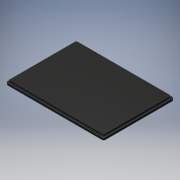
# Autodesk Inventor part: receiver-box-lid
Saved by Autodesk Inventor 2017 (Build 210142000, 142)
## iProperties
Created: 2020-06-15
Part Number: receiver-box-lid
Material: ABS Plastic
Document SubType Name: Modeling
Designer: HAYNIE R&D
Density: 1.06 g/cm^3
Appearance: Glossy - Black
Author: HAYNIE R&D
Autodesk Inventor part; units mm, degrees
(part 1 of 2)
ref_plane "YZ Plane" through (0, 0, 0) normal (1, 0, 0) x (0, 1, 0)
ref_plane "XZ Plane" through (0, 0, 0) normal (0, 1, 0) x (-1, 0, 0)
ref_plane "XY Plane" through (0, 0, 0) normal (0, 0, 1) x (1, 0, 0)
sketch "Sketch2" plane through (0, 0, 0) normal (0, 1, 0) x (-1, 0, 0)
  line L0 (0.0012, 0.0002) -> (-124.9988, 0.0002)
  line L1 (-124.9988, 0.0002) -> (-124.9988, -89.9998)
  line L2 (-124.9988, -89.9998) -> (0.0012, -89.9998)
  line L3 (0.0012, -89.9998) -> (0.0012, 0.0002)
  point P0 (0, 0)
  dimension "d1" = 125
  dimension "d2" = 90
  constraints: 8 end point, 2 parallel, 1 horizontal, 1 perpendicular
  measures "d1" distance of L2.end L1.end
  measures "d2" distance of L1.end L0.end
extrude "Extrusion1" add sketch "Sketch2" along normal blind 2.5
sketch "Sketch3" plane through (0, 2.5, 0) normal (0, 1, 0) x (1, 0, 0)
  line L0 (1.9988, 87.9998) -> (122.9988, 87.9998)
  line L1 (122.9988, 87.9998) -> (122.9988, 1.9998)
  line L2 (122.9988, 1.9998) -> (1.9988, 1.9998)
  line L3 (1.9988, 1.9998) -> (1.9988, 87.9998)
  line L4 (-0.0012, -0.0002) -> (124.9988, -0.0002) projected
  line L5 (124.9988, 89.9998) -> (-0.0012, 89.9998) projected
  line L6 (124.9988, -0.0002) -> (124.9988, 89.9998) projected
  line L7 (-0.0012, 89.9998) -> (-0.0012, -0.0002) projected
  point P0 (0, 0)
  dimension "d13" = 2
  dimension "d14" = 2
  dimension "d15" = 2
  dimension "d16" = 2
  constraints: 8 end point, 2 parallel, 1 horizontal, 1 perpendicular
  measures "d13" distance between parallel lines of L4 L2
  measures "d14" distance between parallel lines of L5 L0
  measures "d15" distance between parallel lines of L1 L6
  measures "d16" distance between parallel lines of L7 L3
extrude "Extrusion2" add sketch "Sketch3" along normal blind 2.5 contours L0 L1 L2 L3
fillet "Fillet1" radius 2 1 edges at (-0.0012, 1.25, 0.0002)
fillet "Fillet2" radius 2 1 edges at (124.9988, 1.25, 0.0002)
fillet "Fillet3" radius 2 1 edges at (124.9988, 1.25, -89.9998)
fillet "Fillet4" radius 2 1 edges at (-0.0012, 1.25, -89.9998)
fillet "Fillet5" radius 2 1 edges at (122.9988, 3.75, -1.9998)
fillet "Fillet6" radius 2 1 edges at (122.9988, 3.75, -87.9998)
fillet "Fillet7" radius 2 1 edges at (1.9988, 3.75, -87.9998)
sketch "Sketch4" plane through (0, 0, 0) normal (0, -1, 0) x (1, 0, 0)
  line L0 (-6.3841, 4.5799) -> (131.1521, 4.5799) construction
  line L1 (131.1521, 4.5799) -> (131.1521, -94.6516) construction
  line L2 (131.1521, -94.6516) -> (-6.3841, -94.6516) construction
  line L3 (-6.3841, -94.6516) -> (-6.3841, 4.5799) construction
  line L4 (20.0195, -41.0232) -> (19.5544, -41.0232)
  line L5 (19.5544, -41.0232) -> (19.5544, -39.3101)
  line L6 (19.5544, -39.3101) -> (17.9434, -39.3101)
  line L7 (17.9434, -39.3101) -> (17.9434, -41.0232)
  line L8 (17.9434, -41.0232) -> (17.4782, -41.0232)
  line L9 (17.4782, -41.0232) -> (17.4782, -37.5232)
  line L10 (17.4782, -37.5232) -> (17.9434, -37.5232)
  line L11 (17.9434, -37.5232) -> (17.9434, -38.896)
  line L12 (17.9434, -38.896) -> (19.5544, -38.896)
  line L13 (19.5544, -38.896) -> (19.5544, -37.5232)
  line L14 (19.5544, -37.5232) -> (20.0195, -37.5232)
  line L15 (20.0195, -37.5232) -> (20.0195, -41.0232)
  line L16 (20.3514, -41.0232) -> (21.5313, -37.5232)
  line L17 (21.5313, -37.5232) -> (22.1042, -37.5232)
  line L18 (22.1042, -37.5232) -> (23.2841, -41.0232)
  line L19 (23.2841, -41.0232) -> (22.7934, -41.0232)
  line L20 (22.7934, -41.0232) -> (22.4758, -40.0447)
  line L21 (22.4758, -40.0447) -> (21.1399, -40.0447)
  line L22 (21.1399, -40.0447) -> (20.8222, -41.0232)
  line L23 (20.8222, -41.0232) -> (20.3514, -41.0232)
  line L24 (22.3481, -39.6476) -> (21.8064, -37.9997)
  line L25 (21.8064, -37.9997) -> (21.2675, -39.6476)
  line L26 (21.2675, -39.6476) -> (22.3481, -39.6476)
  line L27 (26.0665, -37.5232) -> (24.8838, -39.4746)
  line L28 (24.8838, -39.4746) -> (24.8838, -41.0232)
  line L29 (24.8838, -41.0232) -> (24.4187, -41.0232)
  line L30 (24.4187, -41.0232) -> (24.4187, -39.5228)
  line L31 (24.4187, -39.5228) -> (23.2359, -37.5232)
  line L32 (23.2359, -37.5232) -> (23.7521, -37.5232)
  line L33 (23.7521, -37.5232) -> (24.6541, -39.0633)
  line L34 (24.6541, -39.0633) -> (25.573, -37.5232)
  line L35 (25.573, -37.5232) -> (26.0665, -37.5232)
  line L36 (28.8943, -41.0232) -> (28.3725, -41.0232)
  line L37 (28.3725, -41.0232) -> (26.8238, -38.0054)
  line L38 (26.8238, -38.0054) -> (26.8238, -41.0232)
  line L39 (26.8238, -41.0232) -> (26.3899, -41.0232)
  line L40 (26.3899, -41.0232) -> (26.3899, -37.5232)
  line L41 (26.3899, -37.5232) -> (27.0507, -37.5232)
  line L42 (27.0507, -37.5232) -> (28.4604, -40.2943)
  line L43 (28.4604, -40.2943) -> (28.4604, -37.5232)
  line L44 (28.4604, -37.5232) -> (28.8943, -37.5232)
  line L45 (28.8943, -37.5232) -> (28.8943, -41.0232)
  line L46 (30.823, -41.0232) -> (29.4673, -41.0232)
  line L47 (29.4673, -41.0232) -> (29.4673, -40.6658)
  line L48 (29.4673, -40.6658) -> (29.9126, -40.6658)
  line L49 (29.9126, -40.6658) -> (29.9126, -37.8806)
  line L50 (29.9126, -37.8806) -> (29.4673, -37.8806)
  line L51 (29.4673, -37.8806) -> (29.4673, -37.5232)
  line L52 (29.4673, -37.5232) -> (30.823, -37.5232)
  line L53 (30.823, -37.5232) -> (30.823, -37.8806)
  line L54 (30.823, -37.8806) -> (30.3777, -37.8806)
  line L55 (30.3777, -37.8806) -> (30.3777, -40.6658)
  line L56 (30.3777, -40.6658) -> (30.823, -40.6658)
  line L57 (30.823, -40.6658) -> (30.823, -41.0232)
  line L58 (31.3988, -41.0232) -> (31.3988, -37.5232)
  line L59 (31.3988, -37.5232) -> (33.5884, -37.5232)
  line L60 (33.5884, -37.5232) -> (33.5884, -37.9373)
  line L61 (33.5884, -37.9373) -> (31.8639, -37.9373)
  line L62 (31.8639, -37.9373) -> (31.8639, -38.896)
  line L63 (31.8639, -38.896) -> (33.4721, -38.896)
  line L64 (33.4721, -38.896) -> (33.4721, -39.3101)
  line L65 (33.4721, -39.3101) -> (31.8639, -39.3101)
  line L66 (31.8639, -39.3101) -> (31.8639, -40.6091)
  line L67 (31.8639, -40.6091) -> (33.5884, -40.6091)
  line L68 (33.5884, -40.6091) -> (33.5884, -41.0232)
  line L69 (33.5884, -41.0232) -> (31.3988, -41.0232)
  line L70 (38.3109, -41.0232) -> (37.7067, -41.0232)
  line L71 (37.7067, -41.0232) -> (36.6006, -39.6306)
  line L72 (36.6006, -39.6306) -> (36.0674, -39.6306)
  line L73 (36.0674, -39.6306) -> (36.0674, -41.0232)
  line L74 (36.0674, -41.0232) -> (35.6022, -41.0232)
  line L75 (35.6022, -41.0232) -> (35.6022, -37.5232)
  line L76 (35.6022, -37.5232) -> (36.5041, -37.5232)
  spline S0 degree 2 poles (36.5041, -37.5232) (36.8048, -37.5232) (37.2104, -37.5884) (37.3947, -37.7075) knots 0 0 0 1 2 2 2
  spline S1 degree 2 poles (37.3947, -37.7075) (37.5791, -37.8267) (37.7918, -38.1982) (37.7918, -38.4733) knots 0 0 0 1 2 2 2
  spline S2 degree 2 poles (37.7918, -38.4733) (37.7918, -38.8562) (37.4004, -39.3753) (37.0657, -39.5001) knots 0 0 0 1 2 2 2
  line L77 (37.0657, -39.5001) -> (38.3109, -41.0232)
  spline S3 degree 2 poles (37.3068, -38.5102) (37.3068, -38.3571) (37.199, -38.1216) (37.0856, -38.0451) knots 0 0 0 1 2 2 2
  spline S4 degree 2 poles (37.0856, -38.0451) (36.9863, -37.9798) (36.7225, -37.9259) (36.5297, -37.9259) knots 0 0 0 1 2 2 2
  line L78 (36.5297, -37.9259) -> (36.0674, -37.9259)
  line L79 (36.0674, -37.9259) -> (36.0674, -39.242)
  line L80 (36.0674, -39.242) -> (36.4758, -39.242)
  spline S5 degree 2 poles (36.4758, -39.242) (36.6772, -39.242) (36.9977, -39.1711) (37.1083, -39.0605) knots 0 0 0 1 2 2 2
  spline S6 degree 2 poles (37.1083, -39.0605) (37.2104, -38.964) (37.3068, -38.6917) (37.3068, -38.5102) knots 0 0 0 1 2 2 2
  line L81 (38.5888, -41.0232) -> (38.5888, -37.5232)
  line L82 (38.5888, -37.5232) -> (40.7785, -37.5232)
  line L83 (40.7785, -37.5232) -> (40.7785, -37.9373)
  line L84 (40.7785, -37.9373) -> (39.054, -37.9373)
  line L85 (39.054, -37.9373) -> (39.054, -38.896)
  line L86 (39.054, -38.896) -> (40.6622, -38.896)
  line L87 (40.6622, -38.896) -> (40.6622, -39.3101)
  line L88 (40.6622, -39.3101) -> (39.054, -39.3101)
  line L89 (39.054, -39.3101) -> (39.054, -40.6091)
  line L90 (39.054, -40.6091) -> (40.7785, -40.6091)
  line L91 (40.7785, -40.6091) -> (40.7785, -41.0232)
  line L92 (40.7785, -41.0232) -> (38.5888, -41.0232)
  spline S7 degree 2 poles (42.2647, -41.0856) (41.8846, -41.0856) (41.3514, -40.9267) (41.116, -40.8133) knots 0 0 0 1 2 2 2
  line L93 (41.116, -40.8133) -> (41.116, -40.229)
  line L94 (41.116, -40.229) -> (41.15, -40.229)
  spline S8 degree 2 poles (41.15, -40.229) (41.3798, -40.4446) (41.9612, -40.6828) (42.2306, -40.6828) knots 0 0 0 1 2 2 2
  spline S9 degree 2 poles (42.2306, -40.6828) (42.6164, -40.6828) (43.0106, -40.3623) (43.0106, -40.0985) knots 0 0 0 1 2 2 2
  spline S10 degree 2 poles (43.0106, -40.0985) (43.0106, -39.8887) (42.8036, -39.6277) (42.5795, -39.5625) knots 0 0 0 1 2 2 2
  spline S11 degree 2 poles (42.5795, -39.5625) (42.4178, -39.5171) (42.1484, -39.4547) (41.947, -39.4037) knots 0 0 0 1 2 2 2
  spline S12 degree 2 poles (41.947, -39.4037) (41.7655, -39.3554) (41.479, -39.2108) (41.3684, -39.0945) knots 0 0 0 1 2 2 2
  spline S13 degree 2 poles (41.3684, -39.0945) (41.2606, -38.9782) (41.1415, -38.6662) (41.1415, -38.462) knots 0 0 0 1 2 2 2
  spline S14 degree 2 poles (41.1415, -38.462) (41.1415, -38.0366) (41.8052, -37.4608) (42.3186, -37.4608) knots 0 0 0 1 2 2 2
  spline S15 degree 2 poles (42.3186, -37.4608) (42.6135, -37.4608) (43.1354, -37.5771) (43.3595, -37.6877) knots 0 0 0 1 2 2 2
  line L95 (43.3595, -37.6877) -> (43.3595, -38.2436)
  line L96 (43.3595, -38.2436) -> (43.3255, -38.2436)
  spline S16 degree 2 poles (43.3255, -38.2436) (43.1581, -38.0904) (42.6362, -37.8635) (42.3498, -37.8635) knots 0 0 0 1 2 2 2
  spline S17 degree 2 poles (42.3498, -37.8635) (42.0264, -37.8635) (41.6265, -38.167) (41.6265, -38.4138) knots 0 0 0 1 2 2 2
  spline S18 degree 2 poles (41.6265, -38.4138) (41.6265, -38.635) (41.8619, -38.8988) (42.0832, -38.9584) knots 0 0 0 1 2 2 2
  spline S19 degree 2 poles (42.0832, -38.9584) (42.2306, -38.9981) (42.6589, -39.1002) (42.8007, -39.1427) knots 0 0 0 1 2 2 2
  spline S20 degree 2 poles (42.8007, -39.1427) (43.161, -39.2533) (43.4956, -39.6986) (43.4956, -40.0248) knots 0 0 0 1 2 2 2
  spline S21 degree 2 poles (43.4956, -40.0248) (43.4956, -40.2319) (43.3283, -40.6289) (43.178, -40.7679) knots 0 0 0 1 2 2 2
  spline S22 degree 2 poles (43.178, -40.7679) (43.0106, -40.9211) (42.5852, -41.0856) (42.2647, -41.0856) knots 0 0 0 1 2 2 2
  line L97 (43.9693, -41.0232) -> (43.9693, -37.5232)
  line L98 (43.9693, -37.5232) -> (46.1589, -37.5232)
  line L99 (46.1589, -37.5232) -> (46.1589, -37.9373)
  line L100 (46.1589, -37.9373) -> (44.4345, -37.9373)
  line L101 (44.4345, -37.9373) -> (44.4345, -38.896)
  line L102 (44.4345, -38.896) -> (46.0426, -38.896)
  line L103 (46.0426, -38.896) -> (46.0426, -39.3101)
  line L104 (46.0426, -39.3101) -> (44.4345, -39.3101)
  line L105 (44.4345, -39.3101) -> (44.4345, -40.6091)
  line L106 (44.4345, -40.6091) -> (46.1589, -40.6091)
  line L107 (46.1589, -40.6091) -> (46.1589, -41.0232)
  line L108 (46.1589, -41.0232) -> (43.9693, -41.0232)
  line L109 (46.2922, -41.0232) -> (47.4721, -37.5232)
  line L110 (47.4721, -37.5232) -> (48.0451, -37.5232)
  line L111 (48.0451, -37.5232) -> (49.225, -41.0232)
  line L112 (49.225, -41.0232) -> (48.7343, -41.0232)
  line L113 (48.7343, -41.0232) -> (48.4166, -40.0447)
  line L114 (48.4166, -40.0447) -> (47.0807, -40.0447)
  line L115 (47.0807, -40.0447) -> (46.7631, -41.0232)
  line L116 (46.7631, -41.0232) -> (46.2922, -41.0232)
  line L117 (48.289, -39.6476) -> (47.7473, -37.9997)
  line L118 (47.7473, -37.9997) -> (47.2084, -39.6476)
  line L119 (47.2084, -39.6476) -> (48.289, -39.6476)
  line L120 (52.2655, -41.0232) -> (51.6614, -41.0232)
  line L121 (51.6614, -41.0232) -> (50.5552, -39.6306)
  line L122 (50.5552, -39.6306) -> (50.022, -39.6306)
  line L123 (50.022, -39.6306) -> (50.022, -41.0232)
  line L124 (50.022, -41.0232) -> (49.5568, -41.0232)
  line L125 (49.5568, -41.0232) -> (49.5568, -37.5232)
  line L126 (49.5568, -37.5232) -> (50.4588, -37.5232)
  spline S23 degree 2 poles (50.4588, -37.5232) (50.7594, -37.5232) (51.165, -37.5884) (51.3494, -37.7075) knots 0 0 0 1 2 2 2
  spline S24 degree 2 poles (51.3494, -37.7075) (51.5337, -37.8267) (51.7464, -38.1982) (51.7464, -38.4733) knots 0 0 0 1 2 2 2
  spline S25 degree 2 poles (51.7464, -38.4733) (51.7464, -38.8562) (51.355, -39.3753) (51.0204, -39.5001) knots 0 0 0 1 2 2 2
  line L127 (51.0204, -39.5001) -> (52.2655, -41.0232)
  spline S26 degree 2 poles (51.2614, -38.5102) (51.2614, -38.3571) (51.1537, -38.1216) (51.0402, -38.0451) knots 0 0 0 1 2 2 2
  spline S27 degree 2 poles (51.0402, -38.0451) (50.9409, -37.9798) (50.6772, -37.9259) (50.4843, -37.9259) knots 0 0 0 1 2 2 2
  line L128 (50.4843, -37.9259) -> (50.022, -37.9259)
  line L129 (50.022, -37.9259) -> (50.022, -39.242)
  line L130 (50.022, -39.242) -> (50.4304, -39.242)
  spline S28 degree 2 poles (50.4304, -39.242) (50.6318, -39.242) (50.9523, -39.1711) (51.0629, -39.0605) knots 0 0 0 1 2 2 2
  spline S29 degree 2 poles (51.0629, -39.0605) (51.165, -38.964) (51.2614, -38.6917) (51.2614, -38.5102) knots 0 0 0 1 2 2 2
  spline S30 degree 2 poles (53.9105, -41.0856) (53.5702, -41.0856) (52.9944, -40.8558) (52.7845, -40.6261) knots 0 0 0 1 2 2 2
  spline S31 degree 2 poles (52.7845, -40.6261) (52.5746, -40.3992) (52.3449, -39.7185) (52.3449, -39.276) knots 0 0 0 1 2 2 2
  spline S32 degree 2 poles (52.3449, -39.276) (52.3449, -38.8364) (52.569, -38.184) (52.7817, -37.943) knots 0 0 0 1 2 2 2
  spline S33 degree 2 poles (52.7817, -37.943) (52.9916, -37.7075) (53.5645, -37.4608) (53.9191, -37.4608) knots 0 0 0 1 2 2 2
  spline S34 degree 2 poles (53.9191, -37.4608) (54.0949, -37.4608) (54.4041, -37.5118) (54.5345, -37.5515) knots 0 0 0 1 2 2 2
  spline S35 degree 2 poles (54.5345, -37.5515) (54.648, -37.5884) (54.8834, -37.6934) (54.9997, -37.7558) knots 0 0 0 1 2 2 2
  line L131 (54.9997, -37.7558) -> (54.9997, -38.3173)
  line L132 (54.9997, -38.3173) -> (54.9628, -38.3173)
  spline S36 degree 2 poles (54.9628, -38.3173) (54.9004, -38.2606) (54.7075, -38.1018) (54.5686, -38.0252) knots 0 0 0 1 2 2 2
  spline S37 degree 2 poles (54.5686, -38.0252) (54.4353, -37.9515) (54.1204, -37.8579) (53.9162, -37.8579) knots 0 0 0 1 2 2 2
  spline S38 degree 2 poles (53.9162, -37.8579) (53.6922, -37.8579) (53.2922, -38.0422) (53.1419, -38.2181) knots 0 0 0 1 2 2 2
  spline S39 degree 2 poles (53.1419, -38.2181) (52.9944, -38.3968) (52.8299, -38.9385) (52.8299, -39.276) knots 0 0 0 1 2 2 2
  spline S40 degree 2 poles (52.8299, -39.276) (52.8299, -39.6362) (53.0029, -40.1553) (53.1533, -40.334) knots 0 0 0 1 2 2 2
  spline S41 degree 2 poles (53.1533, -40.334) (53.3007, -40.507) (53.695, -40.6828) (53.9162, -40.6828) knots 0 0 0 1 2 2 2
  spline S42 degree 2 poles (53.9162, -40.6828) (54.1176, -40.6828) (54.4608, -40.5836) (54.5941, -40.5098) knots 0 0 0 1 2 2 2
  spline S43 degree 2 poles (54.5941, -40.5098) (54.7217, -40.4361) (54.9118, -40.2829) (54.9657, -40.229) knots 0 0 0 1 2 2 2
  line L133 (54.9657, -40.229) -> (54.9997, -40.229)
  line L134 (54.9997, -40.229) -> (54.9997, -40.7849)
  spline S44 degree 2 poles (54.9997, -40.7849) (54.8834, -40.8388) (54.6792, -40.9381) (54.5345, -40.9835) knots 0 0 0 1 2 2 2
  spline S45 degree 2 poles (54.5345, -40.9835) (54.3814, -41.0345) (54.1204, -41.0856) (53.9105, -41.0856) knots 0 0 0 1 2 2 2
  line L135 (57.975, -41.0232) -> (57.5098, -41.0232)
  line L136 (57.5098, -41.0232) -> (57.5098, -39.3101)
  line L137 (57.5098, -39.3101) -> (55.8988, -39.3101)
  line L138 (55.8988, -39.3101) -> (55.8988, -41.0232)
  line L139 (55.8988, -41.0232) -> (55.4336, -41.0232)
  line L140 (55.4336, -41.0232) -> (55.4336, -37.5232)
  line L141 (55.4336, -37.5232) -> (55.8988, -37.5232)
  line L142 (55.8988, -37.5232) -> (55.8988, -38.896)
  line L143 (55.8988, -38.896) -> (57.5098, -38.896)
  line L144 (57.5098, -38.896) -> (57.5098, -37.5232)
  line L145 (57.5098, -37.5232) -> (57.975, -37.5232)
  line L146 (57.975, -37.5232) -> (57.975, -41.0232)
  line L147 (63.2278, -41.0232) -> (62.6265, -41.0232)
  line L148 (62.6265, -41.0232) -> (62.1472, -40.5212)
  spline S46 degree 2 poles (62.1472, -40.5212) (61.9089, -40.8275) (61.4041, -41.0969) (61.0836, -41.0969) knots 0 0 0 1 2 2 2
  spline S47 degree 2 poles (61.0836, -41.0969) (60.6099, -41.0969) (59.9916, -40.524) (59.9916, -40.0617) knots 0 0 0 1 2 2 2
  spline S48 degree 2 poles (59.9916, -40.0617) (59.9916, -39.8603) (60.105, -39.5455) (60.1986, -39.4178) knots 0 0 0 1 2 2 2
  spline S49 degree 2 poles (60.1986, -39.4178) (60.2894, -39.2959) (60.5305, -39.1087) (60.6383, -39.0406) knots 0 0 0 1 2 2 2
  spline S50 degree 2 poles (60.6383, -39.0406) (60.4028, -38.8818) (60.1674, -38.5272) (60.1674, -38.2606) knots 0 0 0 1 2 2 2
  spline S51 degree 2 poles (60.1674, -38.2606) (60.1674, -38.0933) (60.3007, -37.8097) (60.4085, -37.7019) knots 0 0 0 1 2 2 2
  spline S52 degree 2 poles (60.4085, -37.7019) (60.522, -37.5913) (60.8822, -37.4494) (61.0949, -37.4494) knots 0 0 0 1 2 2 2
  spline S53 degree 2 poles (61.0949, -37.4494) (61.4863, -37.4494) (61.9798, -37.8607) (61.9798, -38.1755) knots 0 0 0 1 2 2 2
  spline S54 degree 2 poles (61.9798, -38.1755) (61.9798, -38.2918) (61.9203, -38.5386) (61.8437, -38.652) knots 0 0 0 1 2 2 2
  spline S55 degree 2 poles (61.8437, -38.652) (61.7643, -38.7683) (61.5147, -38.9697) (61.3048, -39.0463) knots 0 0 0 1 2 2 2
  line L149 (61.3048, -39.0463) -> (62.1302, -39.8972)
  spline S56 degree 2 poles (62.1302, -39.8972) (62.1614, -39.7043) (62.1755, -39.2505) (62.1755, -38.8846) knots 0 0 0 1 2 2 2
  line L150 (62.1755, -38.8846) -> (62.635, -38.8846)
  line L151 (62.635, -38.8846) -> (62.635, -39.1115)
  spline S57 degree 2 poles (62.635, -39.1115) (62.635, -39.3356) (62.5216, -39.9028) (62.3883, -40.1581) knots 0 0 0 1 2 2 2
  line L152 (62.3883, -40.1581) -> (63.2278, -41.0232)
  line L153 (61.943, -40.3141) -> (60.8623, -39.2079)
  spline S58 degree 2 poles (60.8623, -39.2079) (60.8056, -39.2448) (60.6893, -39.3498) (60.6184, -39.4519) knots 0 0 0 1 2 2 2
  spline S59 degree 2 poles (60.6184, -39.4519) (60.5617, -39.5341) (60.4766, -39.8007) (60.4766, -39.9482) knots 0 0 0 1 2 2 2
  spline S60 degree 2 poles (60.4766, -39.9482) (60.4766, -40.2829) (60.8737, -40.714) (61.2112, -40.714) knots 0 0 0 1 2 2 2
  spline S61 degree 2 poles (61.2112, -40.714) (61.4353, -40.714) (61.7955, -40.524) (61.943, -40.3141) knots 0 0 0 1 2 2 2
  spline S62 degree 2 poles (61.0836, -38.8789) (61.214, -38.8336) (61.387, -38.6832) (61.4353, -38.5953) knots 0 0 0 1 2 2 2
  spline S63 degree 2 poles (61.4353, -38.5953) (61.4778, -38.5131) (61.5204, -38.3287) (61.5204, -38.2209) knots 0 0 0 1 2 2 2
  spline S64 degree 2 poles (61.5204, -38.2209) (61.5204, -37.994) (61.2537, -37.7444) (61.0779, -37.7444) knots 0 0 0 1 2 2 2
  spline S65 degree 2 poles (61.0779, -37.7444) (60.868, -37.7444) (60.6269, -38.028) (60.6269, -38.2379) knots 0 0 0 1 2 2 2
  spline S66 degree 2 poles (60.6269, -38.2379) (60.6269, -38.3315) (60.661, -38.4677) (60.7177, -38.5556) knots 0 0 0 1 2 2 2
  spline S67 degree 2 poles (60.7177, -38.5556) (60.7687, -38.6293) (60.9446, -38.7938) (61.0836, -38.8789) knots 0 0 0 1 2 2 2
  spline S68 degree 2 poles (67.6922, -39.276) (67.6922, -39.7554) (67.3036, -40.5268) (66.9774, -40.7424) knots 0 0 0 1 2 2 2
  spline S69 degree 2 poles (66.9774, -40.7424) (66.7108, -40.9097) (66.1634, -41.0232) (65.7379, -41.0232) knots 0 0 0 1 2 2 2
  line L154 (65.7379, -41.0232) -> (64.9324, -41.0232)
  line L155 (64.9324, -41.0232) -> (64.9324, -37.5232)
  line L156 (64.9324, -37.5232) -> (65.7294, -37.5232)
  spline S70 degree 2 poles (65.7294, -37.5232) (66.2229, -37.5232) (66.7845, -37.6707) (66.9831, -37.8011) knots 0 0 0 1 2 2 2
  spline S71 degree 2 poles (66.9831, -37.8011) (67.3206, -38.0252) (67.6922, -38.7655) (67.6922, -39.276) knots 0 0 0 1 2 2 2
  spline S72 degree 2 poles (67.2071, -39.2703) (67.2071, -38.8676) (66.9405, -38.2975) (66.6768, -38.1358) knots 0 0 0 1 2 2 2
  spline S73 degree 2 poles (66.6768, -38.1358) (66.4896, -38.0252) (66.0669, -37.9259) (65.7521, -37.9259) knots 0 0 0 1 2 2 2
  line L157 (65.7521, -37.9259) -> (65.3976, -37.9259)
  line L158 (65.3976, -37.9259) -> (65.3976, -40.6204)
  line L159 (65.3976, -40.6204) -> (65.7521, -40.6204)
  spline S74 degree 2 poles (65.7521, -40.6204) (66.0613, -40.6204) (66.5293, -40.5212) (66.7193, -40.3879) knots 0 0 0 1 2 2 2
  spline S75 degree 2 poles (66.7193, -40.3879) (66.9632, -40.2233) (67.2071, -39.6788) (67.2071, -39.2703) knots 0 0 0 1 2 2 2
  line L160 (68.197, -41.0232) -> (68.197, -37.5232)
  line L161 (68.197, -37.5232) -> (70.3866, -37.5232)
  line L162 (70.3866, -37.5232) -> (70.3866, -37.9373)
  line L163 (70.3866, -37.9373) -> (68.6622, -37.9373)
  line L164 (68.6622, -37.9373) -> (68.6622, -38.896)
  line L165 (68.6622, -38.896) -> (70.2704, -38.896)
  line L166 (70.2704, -38.896) -> (70.2704, -39.3101)
  line L167 (70.2704, -39.3101) -> (68.6622, -39.3101)
  line L168 (68.6622, -39.3101) -> (68.6622, -40.6091)
  line L169 (68.6622, -40.6091) -> (70.3866, -40.6091)
  line L170 (70.3866, -40.6091) -> (70.3866, -41.0232)
  line L171 (70.3866, -41.0232) -> (68.197, -41.0232)
  line L172 (73.4357, -37.5232) -> (72.2302, -41.0232)
  line L173 (72.2302, -41.0232) -> (71.7282, -41.0232)
  line L174 (71.7282, -41.0232) -> (70.5228, -37.5232)
  line L175 (70.5228, -37.5232) -> (71.022, -37.5232)
  line L176 (71.022, -37.5232) -> (71.992, -40.4304)
  line L177 (71.992, -40.4304) -> (72.962, -37.5232)
  line L178 (72.962, -37.5232) -> (73.4357, -37.5232)
  line L179 (73.7704, -41.0232) -> (73.7704, -37.5232)
  line L180 (73.7704, -37.5232) -> (75.96, -37.5232)
  line L181 (75.96, -37.5232) -> (75.96, -37.9373)
  line L182 (75.96, -37.9373) -> (74.2355, -37.9373)
  line L183 (74.2355, -37.9373) -> (74.2355, -38.896)
  line L184 (74.2355, -38.896) -> (75.8437, -38.896)
  line L185 (75.8437, -38.896) -> (75.8437, -39.3101)
  line L186 (75.8437, -39.3101) -> (74.2355, -39.3101)
  line L187 (74.2355, -39.3101) -> (74.2355, -40.6091)
  line L188 (74.2355, -40.6091) -> (75.96, -40.6091)
  line L189 (75.96, -40.6091) -> (75.96, -41.0232)
  line L190 (75.96, -41.0232) -> (73.7704, -41.0232)
  line L191 (78.4985, -41.0232) -> (76.4705, -41.0232)
  line L192 (76.4705, -41.0232) -> (76.4705, -37.5232)
  line L193 (76.4705, -37.5232) -> (76.9357, -37.5232)
  line L194 (76.9357, -37.5232) -> (76.9357, -40.6091)
  line L195 (76.9357, -40.6091) -> (78.4985, -40.6091)
  line L196 (78.4985, -40.6091) -> (78.4985, -41.0232)
  spline S76 degree 2 poles (81.3404, -37.9231) (81.539, -38.1557) (81.7602, -38.8364) (81.7602, -39.2732) knots 0 0 0 1 2 2 2
  spline S77 degree 2 poles (81.7602, -39.2732) (81.7602, -39.6986) (81.5447, -40.3879) (81.3404, -40.6204) knots 0 0 0 1 2 2 2
  spline S78 degree 2 poles (81.3404, -40.6204) (81.1249, -40.8644) (80.5548, -41.0969) (80.2116, -41.0969) knots 0 0 0 1 2 2 2
  spline S79 degree 2 poles (80.2116, -41.0969) (79.8571, -41.0969) (79.2898, -40.8558) (79.0827, -40.6204) knots 0 0 0 1 2 2 2
  spline S80 degree 2 poles (79.0827, -40.6204) (78.8814, -40.3879) (78.6658, -39.7043) (78.6658, -39.2732) knots 0 0 0 1 2 2 2
  spline S81 degree 2 poles (78.6658, -39.2732) (78.6658, -38.8336) (78.8842, -38.1642) (79.0856, -37.9231) knots 0 0 0 1 2 2 2
  spline S82 degree 2 poles (79.0856, -37.9231) (79.2898, -37.6905) (79.8599, -37.4494) (80.2116, -37.4494) knots 0 0 0 1 2 2 2
  spline S83 degree 2 poles (80.2116, -37.4494) (80.569, -37.4494) (81.1419, -37.699) (81.3404, -37.9231) knots 0 0 0 1 2 2 2
  spline S84 degree 2 poles (81.2752, -39.2732) (81.2752, -38.9272) (81.1249, -38.3911) (80.9887, -38.2152) knots 0 0 0 1 2 2 2
  spline S85 degree 2 poles (80.9887, -38.2152) (80.8498, -38.0337) (80.4584, -37.8522) (80.2144, -37.8522) knots 0 0 0 1 2 2 2
  spline S86 degree 2 poles (80.2144, -37.8522) (79.962, -37.8522) (79.5819, -38.028) (79.4373, -38.2152) knots 0 0 0 1 2 2 2
  spline S87 degree 2 poles (79.4373, -38.2152) (79.2983, -38.3939) (79.1508, -38.9328) (79.1508, -39.2732) knots 0 0 0 1 2 2 2
  spline S88 degree 2 poles (79.1508, -39.2732) (79.1508, -39.9624) (79.7294, -40.6942) (80.2144, -40.6942) knots 0 0 0 1 2 2 2
  spline S89 degree 2 poles (80.2144, -40.6942) (80.6994, -40.6942) (81.2752, -39.9624) (81.2752, -39.2732) knots 0 0 0 1 2 2 2
  spline S90 degree 2 poles (84.4831, -38.5783) (84.4831, -38.8052) (84.3214, -39.2136) (84.1768, -39.3554) knots 0 0 0 1 2 2 2
  spline S91 degree 2 poles (84.1768, -39.3554) (83.9952, -39.5341) (83.5045, -39.7185) (83.1302, -39.7185) knots 0 0 0 1 2 2 2
  line L197 (83.1302, -39.7185) -> (82.7359, -39.7185)
  line L198 (82.7359, -39.7185) -> (82.7359, -41.0232)
  line L199 (82.7359, -41.0232) -> (82.2708, -41.0232)
  line L200 (82.2708, -41.0232) -> (82.2708, -37.5232)
  line L201 (82.2708, -37.5232) -> (83.15, -37.5232)
  spline S92 degree 2 poles (83.15, -37.5232) (83.462, -37.5232) (83.8988, -37.6253) (84.0661, -37.7416) knots 0 0 0 1 2 2 2
  spline S93 degree 2 poles (84.0661, -37.7416) (84.2618, -37.8749) (84.4831, -38.2862) (84.4831, -38.5783) knots 0 0 0 1 2 2 2
  spline S94 degree 2 poles (83.9981, -38.5925) (83.9981, -38.4109) (83.8733, -38.1443) (83.7456, -38.0592) knots 0 0 0 1 2 2 2
  spline S95 degree 2 poles (83.7456, -38.0592) (83.635, -37.9855) (83.34, -37.9259) (83.1216, -37.9259) knots 0 0 0 1 2 2 2
  line L202 (83.1216, -37.9259) -> (82.7359, -37.9259)
  line L203 (82.7359, -37.9259) -> (82.7359, -39.3214)
  line L204 (82.7359, -39.3214) -> (83.0536, -39.3214)
  spline S96 degree 2 poles (83.0536, -39.3214) (83.3372, -39.3214) (83.6861, -39.2306) (83.7995, -39.1115) knots 0 0 0 1 2 2 2
  spline S97 degree 2 poles (83.7995, -39.1115) (83.9045, -39.0066) (83.9981, -38.7598) (83.9981, -38.5925) knots 0 0 0 1 2 2 2
  line L205 (87.9263, -41.0232) -> (87.4612, -41.0232)
  line L206 (87.4612, -41.0232) -> (87.4612, -38.0082)
  line L207 (87.4612, -38.0082) -> (86.5479, -40.0588)
  line L208 (86.5479, -40.0588) -> (86.2643, -40.0588)
  line L209 (86.2643, -40.0588) -> (85.3595, -38.0082)
  line L210 (85.3595, -38.0082) -> (85.3595, -41.0232)
  line L211 (85.3595, -41.0232) -> (84.9255, -41.0232)
  line L212 (84.9255, -41.0232) -> (84.9255, -37.5232)
  line L213 (84.9255, -37.5232) -> (85.5609, -37.5232)
  line L214 (85.5609, -37.5232) -> (86.4345, -39.4717)
  line L215 (86.4345, -39.4717) -> (87.2797, -37.5232)
  line L216 (87.2797, -37.5232) -> (87.9263, -37.5232)
  line L217 (87.9263, -37.5232) -> (87.9263, -41.0232)
  line L218 (88.6354, -41.0232) -> (88.6354, -37.5232)
  line L219 (88.6354, -37.5232) -> (90.8251, -37.5232)
  line L220 (90.8251, -37.5232) -> (90.8251, -37.9373)
  line L221 (90.8251, -37.9373) -> (89.1006, -37.9373)
  line L222 (89.1006, -37.9373) -> (89.1006, -38.896)
  line L223 (89.1006, -38.896) -> (90.7088, -38.896)
  line L224 (90.7088, -38.896) -> (90.7088, -39.3101)
  line L225 (90.7088, -39.3101) -> (89.1006, -39.3101)
  line L226 (89.1006, -39.3101) -> (89.1006, -40.6091)
  line L227 (89.1006, -40.6091) -> (90.8251, -40.6091)
  line L228 (90.8251, -40.6091) -> (90.8251, -41.0232)
  line L229 (90.8251, -41.0232) -> (88.6354, -41.0232)
  line L230 (93.84, -41.0232) -> (93.3182, -41.0232)
  line L231 (93.3182, -41.0232) -> (91.7695, -38.0054)
  line L232 (91.7695, -38.0054) -> (91.7695, -41.0232)
  line L233 (91.7695, -41.0232) -> (91.3356, -41.0232)
  line L234 (91.3356, -41.0232) -> (91.3356, -37.5232)
  line L235 (91.3356, -37.5232) -> (91.9964, -37.5232)
  line L236 (91.9964, -37.5232) -> (93.4061, -40.2943)
  line L237 (93.4061, -40.2943) -> (93.4061, -37.5232)
  line L238 (93.4061, -37.5232) -> (93.84, -37.5232)
  line L239 (93.84, -37.5232) -> (93.84, -41.0232)
  line L240 (95.366, -41.0232) -> (95.366, -37.9373)
  line L241 (95.366, -37.9373) -> (94.1917, -37.9373)
  line L242 (94.1917, -37.9373) -> (94.1917, -37.5232)
  line L243 (94.1917, -37.5232) -> (97.0054, -37.5232)
  line L244 (97.0054, -37.5232) -> (97.0054, -37.9373)
  line L245 (97.0054, -37.9373) -> (95.8311, -37.9373)
  line L246 (95.8311, -37.9373) -> (95.8311, -41.0232)
  line L247 (95.8311, -41.0232) -> (95.366, -41.0232)
  line L248 (98.1796, -40.3538) -> (97.5216, -41.8939)
  line L249 (97.5216, -41.8939) -> (97.1784, -41.8939)
  line L250 (97.1784, -41.8939) -> (97.5925, -40.3538)
  line L251 (97.5925, -40.3538) -> (98.1796, -40.3538)
  line L252 (102.349, -41.0232) -> (100.321, -41.0232)
  line L253 (100.321, -41.0232) -> (100.321, -37.5232)
  line L254 (100.321, -37.5232) -> (100.7862, -37.5232)
  line L255 (100.7862, -37.5232) -> (100.7862, -40.6091)
  line L256 (100.7862, -40.6091) -> (102.349, -40.6091)
  line L257 (102.349, -40.6091) -> (102.349, -41.0232)
  line L258 (104.7428, -41.0232) -> (102.7148, -41.0232)
  line L259 (102.7148, -41.0232) -> (102.7148, -37.5232)
  line L260 (102.7148, -37.5232) -> (103.18, -37.5232)
  line L261 (103.18, -37.5232) -> (103.18, -40.6091)
  line L262 (103.18, -40.6091) -> (104.7428, -40.6091)
  line L263 (104.7428, -40.6091) -> (104.7428, -41.0232)
  spline S98 degree 2 poles (106.4758, -41.0856) (106.1354, -41.0856) (105.5597, -40.8558) (105.3498, -40.6261) knots 0 0 0 1 2 2 2
  spline S99 degree 2 poles (105.3498, -40.6261) (105.1399, -40.3992) (104.9101, -39.7185) (104.9101, -39.276) knots 0 0 0 1 2 2 2
  spline S100 degree 2 poles (104.9101, -39.276) (104.9101, -38.8364) (105.1342, -38.184) (105.3469, -37.943) knots 0 0 0 1 2 2 2
  spline S101 degree 2 poles (105.3469, -37.943) (105.5568, -37.7075) (106.1298, -37.4608) (106.4843, -37.4608) knots 0 0 0 1 2 2 2
  spline S102 degree 2 poles (106.4843, -37.4608) (106.6601, -37.4608) (106.9693, -37.5118) (107.0998, -37.5515) knots 0 0 0 1 2 2 2
  spline S103 degree 2 poles (107.0998, -37.5515) (107.2132, -37.5884) (107.4486, -37.6934) (107.5649, -37.7558) knots 0 0 0 1 2 2 2
  line L264 (107.5649, -37.7558) -> (107.5649, -38.3173)
  line L265 (107.5649, -38.3173) -> (107.528, -38.3173)
  spline S104 degree 2 poles (107.528, -38.3173) (107.4657, -38.2606) (107.2728, -38.1018) (107.1338, -38.0252) knots 0 0 0 1 2 2 2
  spline S105 degree 2 poles (107.1338, -38.0252) (107.0005, -37.9515) (106.6857, -37.8579) (106.4815, -37.8579) knots 0 0 0 1 2 2 2
  spline S106 degree 2 poles (106.4815, -37.8579) (106.2574, -37.8579) (105.8575, -38.0422) (105.7071, -38.2181) knots 0 0 0 1 2 2 2
  spline S107 degree 2 poles (105.7071, -38.2181) (105.5597, -38.3968) (105.3951, -38.9385) (105.3951, -39.276) knots 0 0 0 1 2 2 2
  spline S108 degree 2 poles (105.3951, -39.276) (105.3951, -39.6362) (105.5682, -40.1553) (105.7185, -40.334) knots 0 0 0 1 2 2 2
  spline S109 degree 2 poles (105.7185, -40.334) (105.866, -40.507) (106.2602, -40.6828) (106.4815, -40.6828) knots 0 0 0 1 2 2 2
  spline S110 degree 2 poles (106.4815, -40.6828) (106.6828, -40.6828) (107.026, -40.5836) (107.1593, -40.5098) knots 0 0 0 1 2 2 2
  spline S111 degree 2 poles (107.1593, -40.5098) (107.287, -40.4361) (107.477, -40.2829) (107.5309, -40.229) knots 0 0 0 1 2 2 2
  line L266 (107.5309, -40.229) -> (107.5649, -40.229)
  line L267 (107.5649, -40.229) -> (107.5649, -40.7849)
  spline S112 degree 2 poles (107.5649, -40.7849) (107.4486, -40.8388) (107.2444, -40.9381) (107.0998, -40.9835) knots 0 0 0 1 2 2 2
  spline S113 degree 2 poles (107.0998, -40.9835) (106.9466, -41.0345) (106.6857, -41.0856) (106.4758, -41.0856) knots 0 0 0 1 2 2 2
  line L268 (27.6974, -46.7858) -> (27.6974, -43.6999)
  line L269 (27.6974, -43.6999) -> (26.5232, -43.6999)
  line L270 (26.5232, -43.6999) -> (26.5232, -43.2858)
  line L271 (26.5232, -43.2858) -> (29.3368, -43.2858)
  line L272 (29.3368, -43.2858) -> (29.3368, -43.6999)
  line L273 (29.3368, -43.6999) -> (28.1626, -43.6999)
  line L274 (28.1626, -43.6999) -> (28.1626, -46.7858)
  line L275 (28.1626, -46.7858) -> (27.6974, -46.7858)
  line L276 (29.6913, -46.7858) -> (29.6913, -43.2858)
  line L277 (29.6913, -43.2858) -> (31.881, -43.2858)
  line L278 (31.881, -43.2858) -> (31.881, -43.6999)
  line L279 (31.881, -43.6999) -> (30.1565, -43.6999)
  line L280 (30.1565, -43.6999) -> (30.1565, -44.6586)
  line L281 (30.1565, -44.6586) -> (31.7647, -44.6586)
  line L282 (31.7647, -44.6586) -> (31.7647, -45.0727)
  line L283 (31.7647, -45.0727) -> (30.1565, -45.0727)
  line L284 (30.1565, -45.0727) -> (30.1565, -46.3717)
  line L285 (30.1565, -46.3717) -> (31.881, -46.3717)
  line L286 (31.881, -46.3717) -> (31.881, -46.7858)
  line L287 (31.881, -46.7858) -> (29.6913, -46.7858)
  line L288 (34.4195, -46.7858) -> (32.3915, -46.7858)
  line L289 (32.3915, -46.7858) -> (32.3915, -43.2858)
  line L290 (32.3915, -43.2858) -> (32.8567, -43.2858)
  line L291 (32.8567, -43.2858) -> (32.8567, -46.3717)
  line L292 (32.8567, -46.3717) -> (34.4195, -46.3717)
  line L293 (34.4195, -46.3717) -> (34.4195, -46.7858)
  line L294 (34.7853, -46.7858) -> (34.7853, -43.2858)
  line L295 (34.7853, -43.2858) -> (36.975, -43.2858)
  line L296 (36.975, -43.2858) -> (36.975, -43.6999)
  line L297 (36.975, -43.6999) -> (35.2505, -43.6999)
  line L298 (35.2505, -43.6999) -> (35.2505, -44.6586)
  line L299 (35.2505, -44.6586) -> (36.8587, -44.6586)
  line L300 (36.8587, -44.6586) -> (36.8587, -45.0727)
  line L301 (36.8587, -45.0727) -> (35.2505, -45.0727)
  line L302 (35.2505, -45.0727) -> (35.2505, -46.3717)
  line L303 (35.2505, -46.3717) -> (36.975, -46.3717)
  line L304 (36.975, -46.3717) -> (36.975, -46.7858)
  line L305 (36.975, -46.7858) -> (34.7853, -46.7858)
  line L306 (40.4863, -46.7858) -> (40.0212, -46.7858)
  line L307 (40.0212, -46.7858) -> (40.0212, -43.7708)
  line L308 (40.0212, -43.7708) -> (39.1079, -45.8215)
  line L309 (39.1079, -45.8215) -> (38.8242, -45.8215)
  line L310 (38.8242, -45.8215) -> (37.9195, -43.7708)
  line L311 (37.9195, -43.7708) -> (37.9195, -46.7858)
  line L312 (37.9195, -46.7858) -> (37.4855, -46.7858)
  line L313 (37.4855, -46.7858) -> (37.4855, -43.2858)
  line L314 (37.4855, -43.2858) -> (38.1208, -43.2858)
  line L315 (38.1208, -43.2858) -> (38.9944, -45.2344)
  line L316 (38.9944, -45.2344) -> (39.8396, -43.2858)
  line L317 (39.8396, -43.2858) -> (40.4863, -43.2858)
  line L318 (40.4863, -43.2858) -> (40.4863, -46.7858)
  line L319 (41.1954, -46.7858) -> (41.1954, -43.2858)
  line L320 (41.1954, -43.2858) -> (43.385, -43.2858)
  line L321 (43.385, -43.2858) -> (43.385, -43.6999)
  line L322 (43.385, -43.6999) -> (41.6605, -43.6999)
  line L323 (41.6605, -43.6999) -> (41.6605, -44.6586)
  line L324 (41.6605, -44.6586) -> (43.2687, -44.6586)
  line L325 (43.2687, -44.6586) -> (43.2687, -45.0727)
  line L326 (43.2687, -45.0727) -> (41.6605, -45.0727)
  line L327 (41.6605, -45.0727) -> (41.6605, -46.3717)
  line L328 (41.6605, -46.3717) -> (43.385, -46.3717)
  line L329 (43.385, -46.3717) -> (43.385, -46.7858)
  line L330 (43.385, -46.7858) -> (41.1954, -46.7858)
  line L331 (44.7124, -46.7858) -> (44.7124, -43.6999)
  line L332 (44.7124, -43.6999) -> (43.5382, -43.6999)
  line L333 (43.5382, -43.6999) -> (43.5382, -43.2858)
  line L334 (43.5382, -43.2858) -> (46.3518, -43.2858)
  line L335 (46.3518, -43.2858) -> (46.3518, -43.6999)
  line L336 (46.3518, -43.6999) -> (45.1776, -43.6999)
  line L337 (45.1776, -43.6999) -> (45.1776, -46.7858)
  line L338 (45.1776, -46.7858) -> (44.7124, -46.7858)
  line L339 (49.415, -46.7858) -> (48.8109, -46.7858)
  line L340 (48.8109, -46.7858) -> (47.7047, -45.3932)
  line L341 (47.7047, -45.3932) -> (47.1715, -45.3932)
  line L342 (47.1715, -45.3932) -> (47.1715, -46.7858)
  line L343 (47.1715, -46.7858) -> (46.7063, -46.7858)
  line L344 (46.7063, -46.7858) -> (46.7063, -43.2858)
  line L345 (46.7063, -43.2858) -> (47.6083, -43.2858)
  spline S114 degree 2 poles (47.6083, -43.2858) (47.9089, -43.2858) (48.3145, -43.3511) (48.4989, -43.4702) knots 0 0 0 1 2 2 2
  spline S115 degree 2 poles (48.4989, -43.4702) (48.6832, -43.5893) (48.896, -43.9609) (48.896, -44.236) knots 0 0 0 1 2 2 2
  spline S116 degree 2 poles (48.896, -44.236) (48.896, -44.6189) (48.5046, -45.1379) (48.1699, -45.2627) knots 0 0 0 1 2 2 2
  line L346 (48.1699, -45.2627) -> (49.415, -46.7858)
  spline S117 degree 2 poles (48.411, -44.2729) (48.411, -44.1197) (48.3032, -43.8843) (48.1897, -43.8077) knots 0 0 0 1 2 2 2
  spline S118 degree 2 poles (48.1897, -43.8077) (48.0905, -43.7425) (47.8267, -43.6886) (47.6338, -43.6886) knots 0 0 0 1 2 2 2
  line L347 (47.6338, -43.6886) -> (47.1715, -43.6886)
  line L348 (47.1715, -43.6886) -> (47.1715, -45.0046)
  line L349 (47.1715, -45.0046) -> (47.5799, -45.0046)
  spline S119 degree 2 poles (47.5799, -45.0046) (47.7813, -45.0046) (48.1018, -44.9337) (48.2124, -44.8231) knots 0 0 0 1 2 2 2
  spline S120 degree 2 poles (48.2124, -44.8231) (48.3145, -44.7267) (48.411, -44.4544) (48.411, -44.2729) knots 0 0 0 1 2 2 2
  line L350 (52.1435, -43.2858) -> (50.9608, -45.2372)
  line L351 (50.9608, -45.2372) -> (50.9608, -46.7858)
  line L352 (50.9608, -46.7858) -> (50.4956, -46.7858)
  line L353 (50.4956, -46.7858) -> (50.4956, -45.2854)
  line L354 (50.4956, -45.2854) -> (49.3129, -43.2858)
  line L355 (49.3129, -43.2858) -> (49.8291, -43.2858)
  line L356 (49.8291, -43.2858) -> (50.731, -44.826)
  line L357 (50.731, -44.826) -> (51.65, -43.2858)
  line L358 (51.65, -43.2858) -> (52.1435, -43.2858)
  line L359 (56.6788, -46.7858) -> (56.0746, -46.7858)
  line L360 (56.0746, -46.7858) -> (54.9685, -45.3932)
  line L361 (54.9685, -45.3932) -> (54.4353, -45.3932)
  line L362 (54.4353, -45.3932) -> (54.4353, -46.7858)
  line L363 (54.4353, -46.7858) -> (53.9701, -46.7858)
  line L364 (53.9701, -46.7858) -> (53.9701, -43.2858)
  line L365 (53.9701, -43.2858) -> (54.8721, -43.2858)
  spline S121 degree 2 poles (54.8721, -43.2858) (55.1727, -43.2858) (55.5783, -43.3511) (55.7627, -43.4702) knots 0 0 0 1 2 2 2
  spline S122 degree 2 poles (55.7627, -43.4702) (55.947, -43.5893) (56.1597, -43.9609) (56.1597, -44.236) knots 0 0 0 1 2 2 2
  spline S123 degree 2 poles (56.1597, -44.236) (56.1597, -44.6189) (55.7683, -45.1379) (55.4336, -45.2627) knots 0 0 0 1 2 2 2
  line L366 (55.4336, -45.2627) -> (56.6788, -46.7858)
  spline S124 degree 2 poles (55.6747, -44.2729) (55.6747, -44.1197) (55.5669, -43.8843) (55.4535, -43.8077) knots 0 0 0 1 2 2 2
  spline S125 degree 2 poles (55.4535, -43.8077) (55.3542, -43.7425) (55.0905, -43.6886) (54.8976, -43.6886) knots 0 0 0 1 2 2 2
  line L367 (54.8976, -43.6886) -> (54.4353, -43.6886)
  line L368 (54.4353, -43.6886) -> (54.4353, -45.0046)
  line L369 (54.4353, -45.0046) -> (54.8437, -45.0046)
  spline S126 degree 2 poles (54.8437, -45.0046) (55.0451, -45.0046) (55.3656, -44.9337) (55.4762, -44.8231) knots 0 0 0 1 2 2 2
  spline S127 degree 2 poles (55.4762, -44.8231) (55.5783, -44.7267) (55.6747, -44.4544) (55.6747, -44.2729) knots 0 0 0 1 2 2 2
  line L370 (56.9567, -46.7858) -> (56.9567, -43.2858)
  line L371 (56.9567, -43.2858) -> (59.1464, -43.2858)
  line L372 (59.1464, -43.2858) -> (59.1464, -43.6999)
  line L373 (59.1464, -43.6999) -> (57.4219, -43.6999)
  line L374 (57.4219, -43.6999) -> (57.4219, -44.6586)
  line L375 (57.4219, -44.6586) -> (59.0301, -44.6586)
  line L376 (59.0301, -44.6586) -> (59.0301, -45.0727)
  line L377 (59.0301, -45.0727) -> (57.4219, -45.0727)
  line L378 (57.4219, -45.0727) -> (57.4219, -46.3717)
  line L379 (57.4219, -46.3717) -> (59.1464, -46.3717)
  line L380 (59.1464, -46.3717) -> (59.1464, -46.7858)
  line L381 (59.1464, -46.7858) -> (56.9567, -46.7858)
  spline S128 degree 2 poles (61.8692, -44.3409) (61.8692, -44.5679) (61.7075, -44.9763) (61.5629, -45.1181) knots 0 0 0 1 2 2 2
  spline S129 degree 2 poles (61.5629, -45.1181) (61.3814, -45.2968) (60.8907, -45.4811) (60.5163, -45.4811) knots 0 0 0 1 2 2 2
  line L382 (60.5163, -45.4811) -> (60.1221, -45.4811)
  line L383 (60.1221, -45.4811) -> (60.1221, -46.7858)
  line L384 (60.1221, -46.7858) -> (59.6569, -46.7858)
  line L385 (59.6569, -46.7858) -> (59.6569, -43.2858)
  line L386 (59.6569, -43.2858) -> (60.5362, -43.2858)
  spline S130 degree 2 poles (60.5362, -43.2858) (60.8481, -43.2858) (61.2849, -43.3879) (61.4523, -43.5042) knots 0 0 0 1 2 2 2
  spline S131 degree 2 poles (61.4523, -43.5042) (61.648, -43.6375) (61.8692, -44.0488) (61.8692, -44.3409) knots 0 0 0 1 2 2 2
  spline S132 degree 2 poles (61.3842, -44.3551) (61.3842, -44.1736) (61.2594, -43.907) (61.1318, -43.8219) knots 0 0 0 1 2 2 2
  spline S133 degree 2 poles (61.1318, -43.8219) (61.0212, -43.7482) (60.7262, -43.6886) (60.5078, -43.6886) knots 0 0 0 1 2 2 2
  line L387 (60.5078, -43.6886) -> (60.1221, -43.6886)
  line L388 (60.1221, -43.6886) -> (60.1221, -45.0841)
  line L389 (60.1221, -45.0841) -> (60.4397, -45.0841)
  spline S134 degree 2 poles (60.4397, -45.0841) (60.7234, -45.0841) (61.0722, -44.9933) (61.1857, -44.8742) knots 0 0 0 1 2 2 2
  spline S135 degree 2 poles (61.1857, -44.8742) (61.2906, -44.7692) (61.3842, -44.5225) (61.3842, -44.3551) knots 0 0 0 1 2 2 2
  spline S136 degree 2 poles (64.7878, -43.6858) (64.9863, -43.9183) (65.2075, -44.5991) (65.2075, -45.0358) knots 0 0 0 1 2 2 2
  spline S137 degree 2 poles (65.2075, -45.0358) (65.2075, -45.4613) (64.992, -46.1505) (64.7878, -46.3831) knots 0 0 0 1 2 2 2
  spline S138 degree 2 poles (64.7878, -46.3831) (64.5722, -46.627) (64.0021, -46.8596) (63.6589, -46.8596) knots 0 0 0 1 2 2 2
  spline S139 degree 2 poles (63.6589, -46.8596) (63.3044, -46.8596) (62.7371, -46.6185) (62.5301, -46.3831) knots 0 0 0 1 2 2 2
  spline S140 degree 2 poles (62.5301, -46.3831) (62.3287, -46.1505) (62.1131, -45.467) (62.1131, -45.0358) knots 0 0 0 1 2 2 2
  spline S141 degree 2 poles (62.1131, -45.0358) (62.1131, -44.5962) (62.3315, -43.9268) (62.5329, -43.6858) knots 0 0 0 1 2 2 2
  spline S142 degree 2 poles (62.5329, -43.6858) (62.7371, -43.4532) (63.3072, -43.2121) (63.6589, -43.2121) knots 0 0 0 1 2 2 2
  spline S143 degree 2 poles (63.6589, -43.2121) (64.0163, -43.2121) (64.5892, -43.4617) (64.7878, -43.6858) knots 0 0 0 1 2 2 2
  spline S144 degree 2 poles (64.7225, -45.0358) (64.7225, -44.6898) (64.5722, -44.1538) (64.4361, -43.9779) knots 0 0 0 1 2 2 2
  spline S145 degree 2 poles (64.4361, -43.9779) (64.2971, -43.7964) (63.9057, -43.6149) (63.6618, -43.6149) knots 0 0 0 1 2 2 2
  spline S146 degree 2 poles (63.6618, -43.6149) (63.4093, -43.6149) (63.0293, -43.7907) (62.8846, -43.9779) knots 0 0 0 1 2 2 2
  spline S147 degree 2 poles (62.8846, -43.9779) (62.7456, -44.1566) (62.5981, -44.6955) (62.5981, -45.0358) knots 0 0 0 1 2 2 2
  spline S148 degree 2 poles (62.5981, -45.0358) (62.5981, -45.7251) (63.1768, -46.4568) (63.6618, -46.4568) knots 0 0 0 1 2 2 2
  spline S149 degree 2 poles (63.6618, -46.4568) (64.1468, -46.4568) (64.7225, -45.7251) (64.7225, -45.0358) knots 0 0 0 1 2 2 2
  line L390 (68.4268, -46.7858) -> (67.8226, -46.7858)
  line L391 (67.8226, -46.7858) -> (66.7165, -45.3932)
  line L392 (66.7165, -45.3932) -> (66.1832, -45.3932)
  line L393 (66.1832, -45.3932) -> (66.1832, -46.7858)
  line L394 (66.1832, -46.7858) -> (65.7181, -46.7858)
  line L395 (65.7181, -46.7858) -> (65.7181, -43.2858)
  line L396 (65.7181, -43.2858) -> (66.62, -43.2858)
  spline S150 degree 2 poles (66.62, -43.2858) (66.9207, -43.2858) (67.3263, -43.3511) (67.5106, -43.4702) knots 0 0 0 1 2 2 2
  spline S151 degree 2 poles (67.5106, -43.4702) (67.695, -43.5893) (67.9077, -43.9609) (67.9077, -44.236) knots 0 0 0 1 2 2 2
  spline S152 degree 2 poles (67.9077, -44.236) (67.9077, -44.6189) (67.5163, -45.1379) (67.1816, -45.2627) knots 0 0 0 1 2 2 2
  line L397 (67.1816, -45.2627) -> (68.4268, -46.7858)
  spline S153 degree 2 poles (67.4227, -44.2729) (67.4227, -44.1197) (67.3149, -43.8843) (67.2015, -43.8077) knots 0 0 0 1 2 2 2
  spline S154 degree 2 poles (67.2015, -43.8077) (67.1022, -43.7425) (66.8384, -43.6886) (66.6456, -43.6886) knots 0 0 0 1 2 2 2
  line L398 (66.6456, -43.6886) -> (66.1832, -43.6886)
  line L399 (66.1832, -43.6886) -> (66.1832, -45.0046)
  line L400 (66.1832, -45.0046) -> (66.5917, -45.0046)
  spline S155 degree 2 poles (66.5917, -45.0046) (66.793, -45.0046) (67.1135, -44.9337) (67.2242, -44.8231) knots 0 0 0 1 2 2 2
  spline S156 degree 2 poles (67.2242, -44.8231) (67.3263, -44.7267) (67.4227, -44.4544) (67.4227, -44.2729) knots 0 0 0 1 2 2 2
  line L401 (69.5216, -46.7858) -> (69.5216, -43.6999)
  line L402 (69.5216, -43.6999) -> (68.3473, -43.6999)
  line L403 (68.3473, -43.6999) -> (68.3473, -43.2858)
  line L404 (68.3473, -43.2858) -> (71.161, -43.2858)
  line L405 (71.161, -43.2858) -> (71.161, -43.6999)
  line L406 (71.161, -43.6999) -> (69.9867, -43.6999)
  line L407 (69.9867, -43.6999) -> (69.9867, -46.7858)
  line L408 (69.9867, -46.7858) -> (69.5216, -46.7858)
  line L409 (72.7351, -46.7858) -> (71.3793, -46.7858)
  line L410 (71.3793, -46.7858) -> (71.3793, -46.4285)
  line L411 (71.3793, -46.4285) -> (71.8246, -46.4285)
  line L412 (71.8246, -46.4285) -> (71.8246, -43.6432)
  line L413 (71.8246, -43.6432) -> (71.3793, -43.6432)
  line L414 (71.3793, -43.6432) -> (71.3793, -43.2858)
  line L415 (71.3793, -43.2858) -> (72.7351, -43.2858)
  line L416 (72.7351, -43.2858) -> (72.7351, -43.6432)
  line L417 (72.7351, -43.6432) -> (72.2898, -43.6432)
  line L418 (72.2898, -43.6432) -> (72.2898, -46.4285)
  line L419 (72.2898, -46.4285) -> (72.7351, -46.4285)
  line L420 (72.7351, -46.4285) -> (72.7351, -46.7858)
  line L421 (75.8153, -46.7858) -> (75.2934, -46.7858)
  line L422 (75.2934, -46.7858) -> (73.7448, -43.768)
  line L423 (73.7448, -43.768) -> (73.7448, -46.7858)
  line L424 (73.7448, -46.7858) -> (73.3109, -46.7858)
  line L425 (73.3109, -46.7858) -> (73.3109, -43.2858)
  line L426 (73.3109, -43.2858) -> (73.9717, -43.2858)
  line L427 (73.9717, -43.2858) -> (75.3814, -46.0569)
  line L428 (75.3814, -46.0569) -> (75.3814, -43.2858)
  line L429 (75.3814, -43.2858) -> (75.8153, -43.2858)
  line L430 (75.8153, -43.2858) -> (75.8153, -46.7858)
  spline S157 degree 2 poles (77.9908, -46.8539) (77.6192, -46.8539) (77.0037, -46.627) (76.7825, -46.3973) knots 0 0 0 1 2 2 2
  spline S158 degree 2 poles (76.7825, -46.3973) (76.5613, -46.1647) (76.3259, -45.4783) (76.3259, -45.033) knots 0 0 0 1 2 2 2
  spline S159 degree 2 poles (76.3259, -45.033) (76.3259, -44.6104) (76.5641, -43.941) (76.7853, -43.7028) knots 0 0 0 1 2 2 2
  spline S160 degree 2 poles (76.7853, -43.7028) (76.9981, -43.473) (77.6221, -43.2234) (77.9936, -43.2234) knots 0 0 0 1 2 2 2
  spline S161 degree 2 poles (77.9936, -43.2234) (78.1723, -43.2234) (78.4956, -43.2745) (78.6431, -43.3199) knots 0 0 0 1 2 2 2
  spline S162 degree 2 poles (78.6431, -43.3199) (78.7622, -43.3539) (79.0516, -43.4787) (79.1395, -43.5241) knots 0 0 0 1 2 2 2
  line L431 (79.1395, -43.5241) -> (79.1395, -44.0857)
  line L432 (79.1395, -44.0857) -> (79.0998, -44.0857)
  spline S163 degree 2 poles (79.0998, -44.0857) (79.0118, -44.0091) (78.8275, -43.8701) (78.6573, -43.7907) knots 0 0 0 1 2 2 2
  spline S164 degree 2 poles (78.6573, -43.7907) (78.5155, -43.7198) (78.1496, -43.6262) (77.9397, -43.6262) knots 0 0 0 1 2 2 2
  spline S165 degree 2 poles (77.9397, -43.6262) (77.4349, -43.6262) (76.8109, -44.3863) (76.8109, -45.0188) knots 0 0 0 1 2 2 2
  spline S166 degree 2 poles (76.8109, -45.0188) (76.8109, -45.3705) (76.9754, -45.8981) (77.1314, -46.0796) knots 0 0 0 1 2 2 2
  spline S167 degree 2 poles (77.1314, -46.0796) (77.2817, -46.2611) (77.7071, -46.4512) (77.9738, -46.4512) knots 0 0 0 1 2 2 2
  spline S168 degree 2 poles (77.9738, -46.4512) (78.1695, -46.4512) (78.5609, -46.3944) (78.6942, -46.3377) knots 0 0 0 1 2 2 2
  line L433 (78.6942, -46.3377) -> (78.6942, -45.4329)
  line L434 (78.6942, -45.4329) -> (77.883, -45.4329)
  line L435 (77.883, -45.4329) -> (77.883, -45.0245)
  line L436 (77.883, -45.0245) -> (79.1537, -45.0245)
  line L437 (79.1537, -45.0245) -> (79.1537, -46.5533)
  spline S169 degree 2 poles (79.1537, -46.5533) (79.0657, -46.593) (78.7651, -46.7149) (78.6375, -46.7518) knots 0 0 0 1 2 2 2
  spline S170 degree 2 poles (78.6375, -46.7518) (78.4644, -46.8029) (78.1865, -46.8539) (77.9908, -46.8539) knots 0 0 0 1 2 2 2
  spline S171 degree 2 poles (82.2169, -46.8482) (81.8368, -46.8482) (81.3036, -46.6894) (81.0682, -46.576) knots 0 0 0 1 2 2 2
  line L438 (81.0682, -46.576) -> (81.0682, -45.9917)
  line L439 (81.0682, -45.9917) -> (81.1022, -45.9917)
  spline S172 degree 2 poles (81.1022, -45.9917) (81.3319, -46.2072) (81.9134, -46.4455) (82.1828, -46.4455) knots 0 0 0 1 2 2 2
  spline S173 degree 2 poles (82.1828, -46.4455) (82.5686, -46.4455) (82.9628, -46.125) (82.9628, -45.8612) knots 0 0 0 1 2 2 2
  spline S174 degree 2 poles (82.9628, -45.8612) (82.9628, -45.6513) (82.7558, -45.3904) (82.5317, -45.3251) knots 0 0 0 1 2 2 2
  spline S175 degree 2 poles (82.5317, -45.3251) (82.37, -45.2798) (82.1006, -45.2174) (81.8992, -45.1663) knots 0 0 0 1 2 2 2
  spline S176 degree 2 poles (81.8992, -45.1663) (81.7177, -45.1181) (81.4312, -44.9734) (81.3206, -44.8572) knots 0 0 0 1 2 2 2
  spline S177 degree 2 poles (81.3206, -44.8572) (81.2128, -44.7409) (81.0937, -44.4289) (81.0937, -44.2247) knots 0 0 0 1 2 2 2
  spline S178 degree 2 poles (81.0937, -44.2247) (81.0937, -43.7992) (81.7574, -43.2234) (82.2708, -43.2234) knots 0 0 0 1 2 2 2
  spline S179 degree 2 poles (82.2708, -43.2234) (82.5657, -43.2234) (83.0876, -43.3397) (83.3117, -43.4503) knots 0 0 0 1 2 2 2
  line L440 (83.3117, -43.4503) -> (83.3117, -44.0063)
  line L441 (83.3117, -44.0063) -> (83.2776, -44.0063)
  spline S180 degree 2 poles (83.2776, -44.0063) (83.1103, -43.8531) (82.5884, -43.6262) (82.302, -43.6262) knots 0 0 0 1 2 2 2